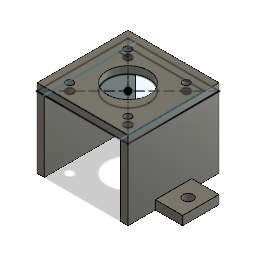
LargeGetShuttleFesting v1 (Autodesk Fusion 360 design; units mm, degrees)
Autodesk Fusion 360 part; units mm, degrees
note: some values were not read from the file. Set by a fixed rule: which sketch regions a step uses.
sketch "Sketch1" plane through (0, 0, 0) normal (0, 1, 0) x (1, 0, 0)
  line L0 (-20.9, 20.9) -> (20.9, 20.9)
  line L1 (20.9, 20.9) -> (20.9, -20.9)
  line L2 (20.9, -20.9) -> (-20.9, -20.9)
  line L3 (-20.9, -20.9) -> (-20.9, 20.9)
  line L4 (-20.9, 20.9) -> (20.9, -20.9) construction
  line L5 (20.9, 20.9) -> (-20.9, -20.9) construction
  line L6 (-20.9, 20.9) -> (-20.9, 16)
  line L7 (-20.9, 16) -> (-16, 16)
  circle A0 centre (-16, 16) radius 2
  circle A1 centre (-16, -16) radius 2
  circle A2 centre (16, -16) radius 2
  circle A3 centre (16, 16) radius 2
  line L8 (-25, 25) -> (25, 25)
  line L9 (25, 25) -> (25, -25)
  line L10 (25, -25) -> (-25, -25)
  line L11 (-25, -25) -> (-25, 25)
  line L12 (-25, 25) -> (25, -25) construction
  line L13 (25, 25) -> (-25, -25) construction
  line L14 (-20.9, 25) -> (-20.9, -25)
  line L15 (20.9, -25) -> (20.9, 25)
  circle A4 centre (0, 0) radius 11.4
  dimension "d1" = 41.8
  dimension "d2" = 41.8
  dimension "d3" = 4.9
  dimension "d4" = 4.9
  dimension "d5" = 4
  dimension "d7" = 360
  dimension "d8" = 50
  dimension "d9" = 50
  dimension "d10" = 22.8
  constraint horizontal L0
  constraint perpendicular L0 L1
  constraint parallel L0 L2
  constraint parallel L1 L3
  constraint coincident L4 A4.centre
  constraint coincident L5 A4.centre
  constraint coincident A4.centre origin
  constraint perpendicular L0 L6
  constraint perpendicular L6 L7
  constraint coincident L7.end A0.centre
  constraint horizontal L8
  constraint perpendicular L8 L9
  constraint parallel L8 L10
  constraint parallel L9 L11
  constraint coincident L12 A4.centre
  constraint coincident L13 A4.centre
  constraint coincident L8 L14.start
  constraint coincident L10 L14.end
  constraint perpendicular L10 L14
  constraint coincident L10 L15.start
  constraint coincident L8 L15.end
  constraint perpendicular L8 L15
  measures "d1" distance of L1.end L2.end
  measures "d2" distance of L0.end L1.end
  measures "d3" distance of L0.start L6.end
  measures "d4" distance of L6.end L7.end
  measures "d5" diameter of A0
  measures "d8" distance of L9.end L10.end
  measures "d9" distance of L8.end L9.end
  measures "d10" diameter of A4
extrude "Extrude1" add sketch "Sketch1" along normal blind 4
extrude "Extrude2" add sketch "Sketch1" against normal blind 39.1 contours L3 L6 L8 L10 L11 L14 | L1 L8 L9 L10 L15
sketch "Sketch2" plane through (-25, 0, 0) normal (-1, 0, 0) x (0, 0, 1)
  line L0 (25, -39.1) -> (25, 4)
  line L1 (25, 4) -> (-25, 4)
  line L2 (-25, 4) -> (-25, -39.1)
  line L3 (-25, -39.1) -> (25, -39.1)
  line L4 (0, -39.1) -> (-10, -39.1)
  line L5 (-10, -39.1) -> (10, -39.1)
  line L6 (10, -39.1) -> (10, -34.1)
  line L7 (10, -34.1) -> (-10, -34.1)
  line L8 (-10, -34.1) -> (-10, -39.1)
  dimension "d15" = 10
  dimension "d16" = 20
  dimension "d17" = 5
  constraint midpoint L3 L4.start
  constraint parallel L3 L4
  constraint horizontal L5
  constraint vertical L6
  constraint horizontal L7
  constraint vertical L8
  measures "d15" distance of L4.start L4.end
  measures "d16" distance of L4.end L5.end
  measures "d17" distance of L4.end L7.end
sketch "Sketch3" plane through (25, 0, 0) normal (1, 0, 0) x (0, 0, -1)
  line L0 (25, -39.1) -> (25, 4)
  line L1 (25, 4) -> (-25, 4)
  line L2 (-25, 4) -> (-25, -39.1)
  line L3 (-25, -39.1) -> (25, -39.1)
  line L4 (0, -39.1) -> (-10, -39.1)
  line L5 (-10, -39.1) -> (10, -39.1)
  line L6 (10, -39.1) -> (10, -34.1)
  line L7 (10, -34.1) -> (-10, -34.1)
  line L8 (-10, -34.1) -> (-10, -39.1)
  dimension "d18" = 20
  dimension "d19" = 5
  constraint midpoint L3 L4.start
  constraint coincident L3 L4.end
  constraint parallel L3 L4
  constraint horizontal L5
  constraint vertical L6
  constraint horizontal L7
  constraint vertical L8
  measures "d18" distance of L4.end L5.end
  measures "d19" distance of L4.end L7.end
extrude "Extrude3" add sketch "Sketch3" along normal blind 15 contours L3 L4 L5 L6 L7 L8
extrude "Extrude4" add sketch "Sketch2" along normal blind 15 contours L3 L4 L5 L6 L7 L8
sketch "Sketch4" plane through (0, -34.1, 0) normal (0, 1, 0) x (-1, 0, 0)
  line L0 (25, 10) -> (25, -10)
  line L1 (25, -10) -> (40, -10)
  line L2 (40, -10) -> (40, 10)
  line L3 (40, 10) -> (25, 10)
  line L4 (40, 0) -> (33, 0)
  circle A0 centre (33, 0) radius 2.8
  dimension "d24" = 7
  dimension "d25" = 5.6
  constraint midpoint L2 L4.start
  constraint perpendicular L2 L4
  constraint coincident L4.end A0.centre
  measures "d24" distance of L4.start L4.end
  measures "d25" diameter of A0
sketch "Sketch5" plane through (0, -34.1, 0) normal (0, 1, 0) x (-1, 0, 0)
  line L0 (-25, -10) -> (-25, 10)
  line L1 (-25, 10) -> (-40, 10)
  line L2 (-40, 10) -> (-40, -10)
  line L3 (-40, -10) -> (-25, -10)
  line L4 (-40, 0) -> (-33, 0)
  circle A0 centre (-33, 0) radius 2.8
  dimension "d26" = 7
  dimension "d27" = 5.6
  constraint midpoint L2 L4.start
  constraint perpendicular L2 L4
  constraint coincident L4.end A0.centre
  measures "d26" distance of L4.start L4.end
  measures "d27" diameter of A0
extrude "Extrude5" cut sketch "Sketch4" sketch "Sketch5" against normal blind 30 contours A0 of sketch 2 contours A0
